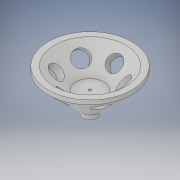
# Autodesk Inventor part: rotor
Saved by Autodesk Inventor 2019.4 (Build 234330000, 330)
## iProperties
Created: 2019-10-31
Part Number: rotor
Material: Genérico
Document SubType Name: Modeling
Designer: natha
Density: 1 g/cm^3
Appearance: Padrão
Author: natha
Autodesk Inventor part; units mm, degrees
ref_plane "YZ Plane" through (0, 0, 0) normal (1, 0, 0) x (0, 1, 0)
ref_plane "XZ Plane" through (0, 0, 0) normal (0, 1, 0) x (-1, 0, 0)
sketch "Esboço1" plane through (0, 0, 0) normal (0, 1, 0) x (-1, 0, 0)
  point P0 (0, 0)
sketch "Esboço2" plane through (0, 0, 0) normal (0, 0, 1) x (1, 0, 0)
  line L0 (0, 0) -> (-5, 0) construction
  line L1 (-5, 0) -> (-5, 3) construction
  line L2 (0, 0) -> (0, 27) construction
  line L3 (0, 27) -> (-30, 27) construction
  line L4 (-30, 27) -> (-30, 30) construction
  line L5 (-5, 3) -> (-30, 27) construction
  line L6 (-30, 30) -> (0, 30) construction
  line L7 (0, 30) -> (0, 27) construction
  line L8 (0, 0) -> (0, 15) construction
  line L9 (0, 15) -> (-10, 15) construction
  line L10 (-10, 15) -> (-25.625, 30) construction
  line L11 (-30, 30) -> (-25.625, 30)
  line L12 (-10, 15) -> (0, 15)
  line L13 (0, 0) -> (-5, 0)
  line L14 (-5, 3) -> (-5, 0)
  line L15 (-5, 3) -> (-30, 27)
  line L16 (-30, 30) -> (-30, 27)
  line L17 (0, 0) -> (0, 15)
  line L18 (-25.625, 30) -> (-10, 15)
  dimension "d0" = 5
  dimension "d1" = 3
  dimension "d2" = 27
  dimension "d3" = 30
  dimension "d4" = 3
  dimension "d5" = 15
  dimension "d6" = 10
  constraints: 38 end point, 5 collinear, 5 perpendicular, 2 horizontal, 2 point on line, 2 vertical, 1 parallel
  measures "d0" distance of L0.start L0.end
  measures "d1" distance of L0.end L1.end
  measures "d2" distance of L0.start L2.end
  measures "d3" distance of L2.end L3.end
  measures "d4" distance of L3.end L4.end
  measures "d5" distance of L0.start L8.end
  measures "d6" distance of L8.end L9.end
revolve "Revolução1" add sketch "Esboço2" angle 360 about axis through (0, 0, 0) along (0, 1, 0)
sketch "Esboço3" plane through (0, 0, 0) normal (1, 0, 0) x (0, 1, 0)
  line L0 (30, -25.625) -> (30, 25.625) projected
  line L1 (15, -10) -> (15, 10) projected
  line L2 (30, 25.625) -> (15, 10)
  point P0 (0, 0)
  constraints: 2 end point
ref_plane "Plano de trabalho1" through (0, 30, 25.625) normal (0, -0.7214, 0.6925) x (1, 0, 0)
sketch "Esboço4" plane through (0, 30, 25.625) normal (0, -0.7214, 0.6925) x (1, 0, 0)
  ellipse E0 centre (0, -28.8735) end of major axis (10, -28.8735) minor radius 7.2139 construction
  ellipse E1 centre (0, -18.4856) end of major axis (25.625, -18.4856) minor radius 18.4856 construction
  line L0 (0, 0) -> (0, -21.6597) construction
  line L1 (0, 0) -> (0, -10.8298) construction
  circle A0 centre (0, -10.8298) radius 5.5
  point P0 (0, -39.2615)
  dimension "d9" = 11
  constraints: 4 end point, 2 vertical alignment, 1 centre point, 1 coincident, 1 midpoint, 1 vertical, 2 other
  measures "d9" diameter of A0
extrude "Extrusão1" cut sketch "Esboço4" along normal blind 10 and the other way blind 5
pattern_circular "Padrão circular1" count 6 over 360 about axis through (0, -10, 0) along (0, 1, 0) of "Extrusão1"
sketch "Esboço5" plane through (0, 0, 0) normal (0, -1, 0) x (1, 0, 0)
  circle A0 centre (0, 0) radius 1
  dimension "d17" = 2
  constraints: 1 centre point, 1 coincident
  measures "d17" diameter of A0
extrude "Extrusão2" cut sketch "Esboço5" against normal up to next
